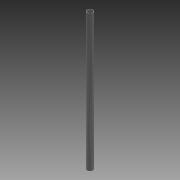
# Autodesk Inventor part: stand_topPole
Saved by Autodesk Inventor 2013 (Build 170138000, 138)
## iProperties
Created: 2013-07-14
Part Number: stand_topPole
Material: Steel, Alloy
Document SubType Name: Modeling
Designer: David DeBoer
Mass: 3685.66 g
Surface Area: 3704.64 cm^2
Volume: 469.511 cm^3
Density: 7.85 g/cm^3
Company: HERA Project
Author: David DeBoer
Autodesk Inventor part; units mm, degrees
ref_plane "YZ Plane" through (0, 0, 0) normal (1, 0, 0) x (0, 1, 0)
ref_plane "XZ Plane" through (0, 0, 0) normal (0, 1, 0) x (-1, 0, 0)
ref_plane "XY Plane" through (0, 0, 0) normal (0, 0, 1) x (1, 0, 0)
sketch "Sketch1" plane through (0, 0, 0) normal (0, 1, 0) x (-1, 0, 0)
  circle A0 centre (0, 0) radius 25.4
  circle A1 centre (0, 0) radius 22.86
  dimension "d0" = 50.8
  dimension "d2" = 2.54
  constraints: 2 centre point, 1 coincident
  measures "d0" diameter of A0
  measures "d2" radial gap between concentric circles of A1 A0
extrude "Extrusion1" add sketch "Sketch1" along normal blind 1219.2
body "Solid1"
